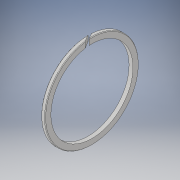
# Autodesk Inventor part: Component 8(Piston Ring)
Saved by Autodesk Inventor 2018 (Build 220112000, 112)
## iProperties
Created: 2023-03-14
Part Number: Component 8(Piston Ring)
Material: Generic
Document SubType Name: Modeling
Designer: Habib Mohamed
Density: 1 g/cm^3
Appearance: Default
Author: Habib Mohamed
Autodesk Inventor part; units mm, degrees
ref_plane "YZ Plane" through (0, 0, 0) normal (1, 0, 0) x (0, 1, 0)
ref_plane "XZ Plane" through (0, 0, 0) normal (0, 1, 0) x (-1, 0, 0)
ref_plane "XY Plane" through (0, 0, 0) normal (0, 0, 1) x (1, 0, 0)
sketch "Sketch1" plane through (0, 0, 0) normal (1, 0, 0) x (0, 1, 0)
  circle A0 centre (0, 0) radius 12
  circle A1 centre (0, 0) radius 10.5
  dimension "d0" = 24
  dimension "d1" = 21
  constraints: 2 centre point, 2 coincident
  measures "d0" diameter of A0
  measures "d1" diameter of A1
extrude "Extrusion1" add sketch "Sketch1" along normal blind 1
sketch "Sketch2" plane through (0, 0, 0) normal (0, 1, 0) x (-1, 0, 0)
  line L0 (-1, 0.73) -> (0, -1.0021)
  line L1 (0, -12) -> (0, 12) projected
  line L2 (0, -12) -> (-1, -12) projected
  line L3 (-1, -12) -> (-1, -10.5) projected
  line L4 (-1, -10.5) -> (0, -10.5) projected
  line L5 (0, -10.5) -> (0, -12) projected
  line L6 (-1, 12) -> (0, 12) projected
  line L7 (0, 12) -> (0, 10.5) projected
  line L8 (0, 10.5) -> (-1, 10.5) projected
  line L9 (-1, 10.5) -> (-1, 12) projected
  line L10 (-1, 1.73) -> (0, -0.0021)
  line L11 (-1, 0.73) -> (-1, 1.73)
  line L12 (-1, 12) -> (-1, -12) projected
  line L13 (0, -1.0021) -> (0, -0.0021)
  point P0 (0, 0)
  dimension "d4" = 12.73
  dimension "d5" = 30
  dimension "d6" = 1
  constraints: 8 end point, 3 point on line, 1 collinear, 1 parallel
  measures "d4" distance from line of L0.start L2
  measures "d5" angle of L1 L0
  measures "d6" distance of L10.start L0.start
extrude "Extrusion2" cut sketch "Sketch2" along normal blind 17 contours L11 L10 L1 L0
fillet "Fillet1" radius 0.15 4 edges at (1, -11.9686, -0.8673) (1, 11.9944, 0.3652) (0, -11.9895, 0.5015) (0, 12, -0.001)
body "Solid1"
